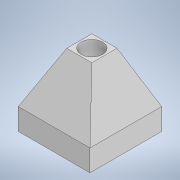
# Autodesk Inventor part: Stand
Saved by Autodesk Inventor 2020 (Build 240168000, 168)
## iProperties
Created: 2021-05-03
Part Number: Stand
Material: Generic
Document SubType Name: Modeling
Designer: chick
Density: 1 g/cm^3
Appearance: Default
Author: chick
Autodesk Inventor part; units mm, degrees
ref_plane "YZ Plane" through (0, 0, 0) normal (1, 0, 0) x (0, 1, 0)
ref_plane "XZ Plane" through (0, 0, 0) normal (0, 1, 0) x (-1, 0, 0)
ref_plane "XY Plane" through (0, 0, 0) normal (0, 0, 1) x (1, 0, 0)
sketch "Sketch3" plane through (0, 0, 0) normal (0, 1, 0) x (-1, 0, 0)
  line L0 (10, 0) -> (10, -10)
  line L1 (10, -10) -> (0, -10)
  line L2 (0, -10) -> (0, 0)
  line L3 (0, 0) -> (10, 0)
  dimension "d0" = 10
  dimension "d1" = 10
  constraints: 8 end point, 3 perpendicular, 1 vertical
  measures "d0" distance of L0.start L0.end
  measures "d1" distance of L0.end L1.end
extrude "Extrusion1" add sketch "Sketch3" along normal blind 10
sketch "Sketch4" plane through (0, 0, 0) normal (1, 0, 0) x (0, 0, -1)
  line L0 (10, 10) -> (0, 10) projected
  line L1 (3.4236, 10) -> (0, 3)
  line L2 (0, 0) -> (0, 10) projected
  line L3 (6.9236, 10) -> (10, 3)
  line L4 (10, 0) -> (10, 10) projected
  line L5 (3.4236, 10) -> (6.9236, 10)
  dimension "d4" = 3.5
  dimension "d5" = 7
  dimension "d6" = 7
  constraints: 6 end point, 4 point on line, 1 collinear
  measures "d4" distance of L3.start L1.start
  measures "d5" distance of L3.end L0.start
  measures "d6" distance of L1.end L0.end
extrude "Extrusion2" cut sketch "Sketch4" against normal blind 10
sketch "Sketch6" plane through (-10, 0, 0) normal (0, 0, 1) x (1, 0, 0)
  line L0 (0, 10) -> (10, 10) projected
  line L1 (3.3385, 10) -> (0, 3)
  line L2 (0, 3) -> (0, 10) projected
  line L3 (3.3385, 10) -> (6.8385, 10)
  line L4 (6.8385, 10) -> (10, 3)
  line L5 (10, 10) -> (10, 3) projected
  point P0 (10, 0)
  dimension "d12" = 3.5
  dimension "d13" = 7
  dimension "d14" = 7
  constraints: 6 end point, 3 point on line, 1 horizontal
  measures "d12" distance of L3.end L1.start
  measures "d13" vertical distance of L4.end L3.end
  measures "d14" vertical distance of L1.end L1.start
extrude "Extrusion3" cut sketch "Sketch6" against normal blind 10
sketch "Sketch7" plane through (0, 10, 0) normal (0, 1, 0) x (1, 0, 0)
  circle A0 centre (-4.9115, 5.1736) radius 1.5
  line L0 (-6.6615, 3.4236) -> (-3.1615, 3.4236) projected
  point P0 (0, 0)
  dimension "d17" = 1.75
  dimension "d18" = 3
  constraints: 1 centre point
  measures "d17" distance from line of A0.centre L0
  measures "d18" diameter of A0
extrude "Extrusion4" cut sketch "Sketch7" against normal blind 10
body "Solid1"
